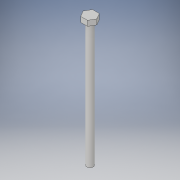
# Autodesk Inventor part: Bag motor bolt
Saved by Autodesk Inventor 2017 (Build 210142000, 142)
## iProperties
Created: 2016-09-26
Part Number: Bag motor bolt
Material: Generic
Document SubType Name: Modeling
Designer: hanso
Density: 1 g/cm^3
Appearance: Default
Author: hanso
Autodesk Inventor part; units mm, degrees
ref_plane "YZ Plane" through (0, 0, 0) normal (1, 0, 0) x (0, 1, 0)
ref_plane "XZ Plane" through (0, 0, 0) normal (0, 1, 0) x (-1, 0, 0)
ref_plane "XY Plane" through (0, 0, 0) normal (0, 0, 1) x (1, 0, 0)
sketch "Sketch1" plane through (0, 0, 0) normal (0, 1, 0) x (-1, 0, 0)
  circle A0 centre (0, 0) radius 1.9844
  dimension "d0" = 3.9688
  constraints: 1 centre point, 1 coincident
  measures "d0" diameter of A0
extrude "Extrusion1" add sketch "Sketch1" along normal blind 76.2
sketch "Sketch2" plane through (0, 76.2, 0) normal (0, 1, 0) x (1, 0, 0)
  line L0 (-4.1682, 0) -> (-2.0841, 3.6098)
  line L1 (-2.0841, 3.6098) -> (2.0841, 3.6098)
  line L2 (2.0841, 3.6098) -> (4.1682, 0)
  line L3 (4.1682, 0) -> (2.0841, -3.6098)
  line L4 (2.0841, -3.6098) -> (-2.0841, -3.6098)
  line L5 (-2.0841, -3.6098) -> (-4.1682, 0)
  point P0 (0, 0)
  point P1 (0, 0)
  constraints: 12 end point, 1 coincident, 13 other
extrude "Extrusion2" add sketch "Sketch2" along normal blind 3.175
body "Solid1"
